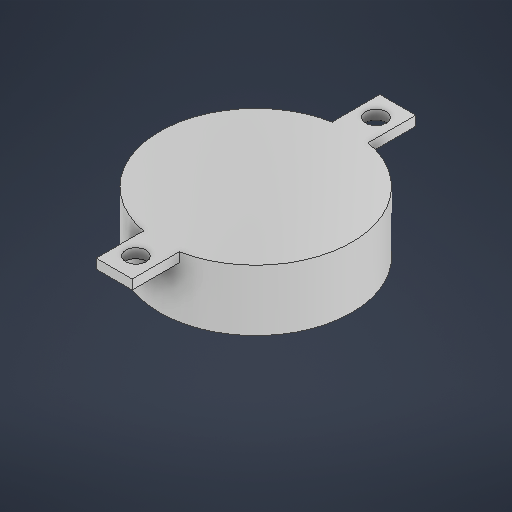
# Autodesk Inventor part: ball_caster
Saved by Autodesk Inventor 2026 (Build 300175050, 175E)
## iProperties
Created: 2025-06-14
Part Number: ball_caster
Material: Generic
Document SubType Name: Modeling
Designer: satom
Density: 1 g/cm^3
Appearance: Default
Author: satom
Autodesk Inventor part; units mm, degrees
ref_plane "YZ Plane" through (0, 0, 0) normal (1, 0, 0) x (0, 1, 0)
ref_plane "XZ Plane" through (0, 0, 0) normal (0, 1, 0) x (-1, 0, 0)
ref_plane "XY Plane" through (0, 0, 0) normal (0, 0, 1) x (1, 0, 0)
sketch "Sketch1" plane through (0, 0, 0) normal (0, 0, 1) x (1, 0, 0)
  line L0 (0, 0) -> (16, 0)
  line L1 (16, 0) -> (16, -10.16)
  line L2 (0, 0) -> (0, -20)
  arc A0 (0, -20) -> (5.3946, -14.6054) centre (0, -14.6054) ccw
  line L3 (0, -14.6054) -> (5.3946, -14.6054) construction
  line L4 (0, -14.6054) -> (0, -20) construction
  line L5 (5.3946, -14.6054) -> (16, -10.16)
  dimension "d0" = 16
  dimension "d1" = 20
  dimension "d2" = 10.16
  dimension "d3" = 90
  dimension "d4" = 5.3946
  constraints: 12 end point, 2 point on circle, 1 centre point, 1 horizontal, 1 perpendicular, 1 point on line, 1 vertical
  measures "d0" distance of L0.start L0.end
  measures "d1" distance of L0.start L2.end
  measures "d2" distance of L0.end L1.end
  measures "d3" angle of L4 L3
  measures "d4" radius of A0
revolve "Revolution1" add sketch "Sketch1" angle 360 about axis through (0, 0, 0) along (0, -1, 0)
sketch "Sketch2" plane through (0, 0, 0) normal (0, 1, 0) x (1, 0, 0)
  circle A0 centre (0, 20.0361) radius 1.7
  circle A1 centre (0, -19.9639) radius 1.7
  line L0 (0, 24.0573) -> (0, -23.8232) construction
  line L1 (-3, 23.6661) -> (-3, 15.7162)
  line L2 (3, 23.6661) -> (3, 15.7162)
  line L3 (-3, 23.6661) -> (3, 23.6661)
  line L4 (-3, -23.5939) -> (-3, -15.7162)
  line L5 (3, -23.5939) -> (3, -15.7162)
  line L6 (-3, -23.5939) -> (3, -23.5939)
  circle A2 centre (0, 0) radius 16 projected
  circle A3 centre (0, 0) radius 16
  dimension "d6" = 3.4
  dimension "d7" = 3.4
  dimension "d8" = 40
  dimension "d10" = 3
  dimension "d11" = 3
  dimension "d12" = 3.63
  dimension "d13" = 3
  dimension "d14" = 3
  dimension "d15" = 3.63
  dimension "d18" = 32
  constraints: 14 end point, 6 vertical, 4 point on circle, 3 centre point, 2 horizontal, 2 point on line, 1 coincident
  measures "d6" diameter of A0
  measures "d7" diameter of A1
  measures "d8" distance of A0.centre A1.centre
  measures "d10" distance from line of A0.centre L2
  measures "d11" distance from line of A0.centre L1
  measures "d12" distance from line of A0.centre L3
  measures "d13" distance from line of A1.centre L4
  measures "d14" distance from line of L5 A1.centre
  measures "d15" distance from line of A1.centre L6
  measures "d18" diameter of A3
extrude "Extrusion1" add sketch "Sketch2" against normal blind 1.5875 contours L3 L2 A2 L1 | A2 L5 L6 L4
equation "\"d6\" = m3_clearance"
equation "\"d7\" = m3_clearance"
equation "\"d13\" = d11"
equation "\"d14\" = d13"
equation "\"d15\" = d12"
equation "\"m3_heat_set_insert\" = 4"
equation "\"m3_clearance\" = 3.4"
equation "\"m3_heat_set_depth\" = 7"
equation "\"robot_diameter\" = 354"
equation "\"hardboard_thickness\" = 5"
equation "\"motor_centerline_height\" = 13"
body "Solid1"
